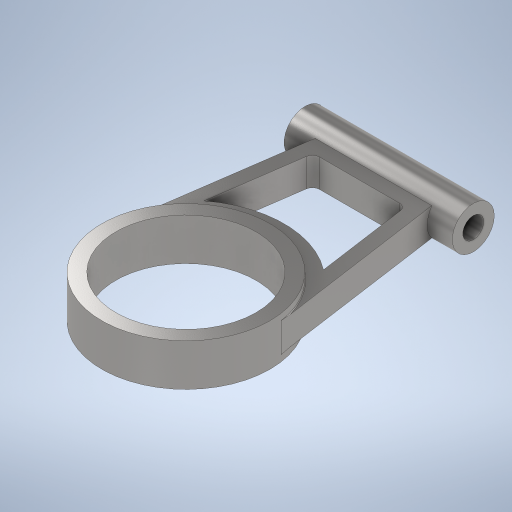
# Autodesk Inventor part: practice5
Saved by Autodesk Inventor 2024 (Build 280153000, 153)
## iProperties
Created: 2024-02-15
Part Number: practice5
Material: Stahl, galvanisiert
Document SubType Name: Modeling
Designer: ffogue
Density: 7.85 g/cm^3
Appearance: Galvanisiert
Author: ffogue
Autodesk Inventor part; units mm, degrees
ref_plane "YZ Plane" through (0, 0, 0) normal (1, 0, 0) x (0, 1, 0)
ref_plane "XZ Plane" through (0, 0, 0) normal (0, 1, 0) x (-1, 0, 0)
ref_plane "XY Plane" through (0, 0, 0) normal (0, 0, 1) x (1, 0, 0)
sketch "Skizze1" plane through (0, 0, 0) normal (0, 0, 1) x (1, 0, 0)
  circle A0 centre (0, 0) radius 50
  circle A1 centre (0, 0) radius 60
  line L0 (-59.4034, 8.4405) -> (-40, 145)
  line L1 (59.4034, 8.4405) -> (40, 145)
  line L2 (-60, 145) -> (60, 145)
  line L3 (0, 0) -> (0, 124.4814) construction
  line L4 (-60, 145) -> (-60, 160)
  line L5 (-60, 160) -> (60, 160)
  line L6 (60, 160) -> (60, 145)
  point P0 (40, 145)
  dimension "d0" = 100
  dimension "d1" = 120
  dimension "d2" = 30
  dimension "d3" = 120
  dimension "d4" = 80
  dimension "d5" = 160
  constraints: 14 end point, 2 centre point, 2 coincident, 2 perpendicular, 2 point on circle, 2 symmetric about line, 2 tangent, 2 vertical, 1 horizontal, 1 point on line
  measures "d0" diameter of A0
  measures "d1" diameter of A1
  measures "d2" diameter of L5 L2
  measures "d3" distance between parallel lines of L6 L4
  measures "d4" distance of L1.end L0.end
  measures "d5" distance from line of point (0, 0) L5
extrude "Extrusion3" add sketch "Skizze1" along normal mid plane 20 contours A1 L0 L2 L1
extrude "Extrusion4" add sketch "Skizze1" along normal mid plane 30 contours A1
revolve "Umdrehung2" add sketch "Skizze1" angle 360 about axis through (-60, 145, 0) along (1, 0, 0) contours L2 L4 L5 L6
sketch "Skizze3" plane through (60, 145, 0) normal (1, 0, 0) x (0, 0, -1)
  circle A0 centre (0, 0) radius 15 projected
  point P0 (0, -145)
  constraints: 1 coincident
hole "Bohrung1" at (60, 145, 0) direction (-1, 0, 0) diameter 15 end through all
sketch "Skizze4" plane through (0, 0, 10) normal (0, 0, 1) x (1, 0, 0)
  arc A0 (42.6112, 55.5363) -> (-42.6112, 55.5363) centre (0, 0) ccw
  line L0 (-42.6112, 55.5363) -> (-32.909, 123.8197)
  line L1 (-32.909, 123.8197) -> (32.909, 123.8197)
  line L2 (32.909, 123.8197) -> (42.6112, 55.5363)
  circle A1 centre (0, 0) radius 60 projected
  circle A2 centre (0, 0) radius 50 projected
  circle A3 centre (0, 0) radius 60 projected
  line L3 (0, 0) -> (0, 36.6234) construction
  line L4 (41.5886, 133.8197) -> (-41.5886, 133.8197) projected
  line L5 (-41.5886, 133.8197) -> (-59.4034, 8.4405) projected
  dimension "d24" = 10
  dimension "d25" = 70
  dimension "d27" = 10
  dimension "d28" = 10
  constraints: 8 end point, 2 point on circle, 1 centre point, 1 concentric, 1 equal length, 1 horizontal, 1 symmetric about line, 1 vertical, 1 other
  measures "d24" distance between parallel lines of L1 L4
  measures "d25" radius of A0
  measures "d27" distance from line of L5 L0.end
  measures "d28" distance from line of L5 L0.start
extrude "Extrusion5" cut sketch "Skizze4" against normal up to surface (20 mm away) contours A0 L0 L1 L2
fillet "Rundung1" radius 5 2 edges at (-32.909, 123.8197, 0) (32.909, 123.8197, 0)
fillet "Rundung2" radius 0.5 1 edges at (0, 60, -10)
fillet "Rundung3" radius 0.5 1 edges at (0, 60, 10)
